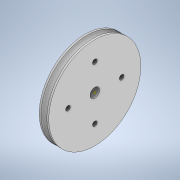
# Autodesk Inventor part: RD0012_ホイール
Saved by Autodesk Inventor 2021.3 (Build 253353000, 353)
## iProperties
Created: 2021-10-14
Part Number: RD0012_ホイール
Material: 一般
Document SubType Name: Modeling
Designer: gilte
Density: 1 g/cm^3
Appearance: 既定
Author: gilte
Autodesk Inventor part; units mm, degrees
ref_plane "YZ Plane" through (0, 0, 0) normal (1, 0, 0) x (0, 1, 0)
ref_plane "XZ Plane" through (0, 0, 0) normal (0, 1, 0) x (-1, 0, 0)
ref_plane "XY Plane" through (0, 0, 0) normal (0, 0, 1) x (1, 0, 0)
sketch "スケッチ1" plane through (0, 0, 0) normal (0, 0, 1) x (1, 0, 0)
  line L0 (0, 0) -> (5, 0)
  line L1 (5, 0) -> (5, 24)
  line L2 (0, 24) -> (0, 0)
  arc A0 (1, 24) -> (4, 24) centre (2.5, 24) ccw
  line L3 (5, 24) -> (4, 24)
  line L4 (1, 24) -> (0, 24)
  dimension "d0" = 5
  dimension "d1" = 24
  dimension "d2" = 3
  constraints: 10 end point, 3 parallel, 2 point on circle, 1 centre point, 1 horizontal, 1 perpendicular
  measures "d0" distance of L2.start L1.end
  measures "d1" distance of L1.end L0.end
  measures "d2" diameter of A0
revolve "回転1" add sketch "スケッチ1" angle 360 about axis through (0, 0, 0) along (1, 0, 0)
sketch "スケッチ2" plane through (5, 0, 0) normal (1, 0, 0) x (0, 0, -1)
  point P0 (0, 0)
hole "穴1" at (5, 0, 0) direction (-1, 0, 0) diameter 5 end through all
sketch "スケッチ3" plane through (5, 0, 0) normal (1, 0, 0) x (0, 0, -1)
  point P0 (0, 0)
  point P1 (0, 14)
  point P2 (-14, 0)
  point P3 (0, -14)
  point P4 (14, 0)
  dimension "d13" = 360
  dimension "d15" = 14
  constraints: 1 vertical alignment, 5 other
  measures "d15" distance of point (14, 0) point (0, 0)
hole "穴2" at (5, 14, 0) at (5, 0, 14) at (5, -14, 0) at (5, 0, -14) direction (-1, 0, 0) diameter 2.459 end through all thread size "M3x0.5" class "6H" standard "ANSI Metric M Profile"
sketch "スケッチ4" plane through (5, 0, 0) normal (1, 0, 0) x (0, 0, -1)
  point P0 (0, 0)
